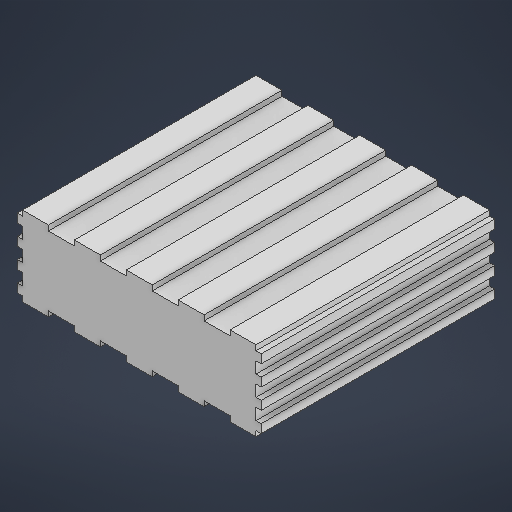
# Autodesk Inventor part: paredBase
Saved by Autodesk Inventor 2026 (Build 300175000, 175)
## iProperties
Created: 2026-04-21
Part Number: paredBase
Material: Generic
Document SubType Name: Modeling
Designer: juana
Density: 1 g/cm^3
Appearance: Default
Author: juana
Autodesk Inventor part; units mm, degrees
ref_plane "YZ Plane" through (0, 0, 0) normal (1, 0, 0) x (0, 1, 0)
ref_plane "XZ Plane" through (0, 0, 0) normal (0, 1, 0) x (-1, 0, 0)
ref_plane "XY Plane" through (0, 0, 0) normal (0, 0, 1) x (1, 0, 0)
sketch "Sketch1" plane through (0, 0, 0) normal (0, 0, 1) x (1, 0, 0)
  line L0 (0, 40) -> (135, 40)
  line L1 (135, 40) -> (135, 0)
  line L2 (135, 0) -> (0, 0)
  line L3 (0, 0) -> (0, 40)
  line L4 (-3, 40) -> (0, 40)
  line L5 (0, 40) -> (0, 35)
  line L6 (0, 35) -> (-3, 35)
  line L7 (-3, 35) -> (-3, 40)
  line L8 (-3, 28.35) -> (0, 28.35)
  line L9 (0, 28.35) -> (0, 23.35)
  line L10 (0, 23.35) -> (-3, 23.35)
  line L11 (-3, 23.35) -> (-3, 28.35)
  line L12 (-3, 16.7) -> (0, 16.7)
  line L13 (0, 16.7) -> (0, 11.7)
  line L14 (0, 11.7) -> (-3, 11.7)
  line L15 (-3, 11.7) -> (-3, 16.7)
  line L16 (135, 40) -> (138, 40)
  line L17 (138, 40) -> (138, 35)
  line L18 (138, 35) -> (135, 35)
  line L19 (135, 35) -> (135, 40)
  line L20 (135, 28.35) -> (138, 28.35)
  line L21 (138, 28.35) -> (138, 23.35)
  line L22 (138, 23.35) -> (135, 23.35)
  line L23 (135, 23.35) -> (135, 28.35)
  line L24 (135, 16.7) -> (138, 16.7)
  line L25 (138, 16.7) -> (138, 11.7)
  line L26 (138, 11.7) -> (135, 11.7)
  line L27 (135, 11.7) -> (135, 16.7)
  line L28 (0, 40) -> (15, 40)
  line L29 (15, 40) -> (15, 43)
  line L30 (15, 43) -> (0, 43)
  line L31 (0, 43) -> (0, 40)
  line L32 (30, 43) -> (30, 40)
  line L33 (30, 40) -> (45, 40)
  line L34 (45, 43) -> (30, 43)
  line L35 (45, 40) -> (45, 43)
  line L36 (60, 43) -> (60, 40)
  line L37 (60, 40) -> (75, 40)
  line L38 (75, 43) -> (60, 43)
  line L39 (75, 40) -> (75, 43)
  line L40 (90, 43) -> (90, 40)
  line L41 (90, 40) -> (105, 40)
  line L42 (105, 43) -> (90, 43)
  line L43 (105, 40) -> (105, 43)
  line L44 (120, 43) -> (120, 40)
  line L45 (120, 40) -> (135, 40)
  line L46 (135, 43) -> (120, 43)
  line L47 (135, 40) -> (135, 43)
  line L48 (0, 0) -> (0, -3)
  line L49 (0, -3) -> (15, -3)
  line L50 (15, 0) -> (0, 0)
  line L51 (15, -3) -> (15, 0)
  line L52 (30, 0) -> (30, -3)
  line L53 (30, -3) -> (45, -3)
  line L54 (45, 0) -> (30, 0)
  line L55 (45, -3) -> (45, 0)
  line L56 (60, 0) -> (60, -3)
  line L57 (60, -3) -> (75, -3)
  line L58 (75, 0) -> (60, 0)
  line L59 (75, -3) -> (75, 0)
  line L60 (90, 0) -> (90, -3)
  line L61 (90, -3) -> (105, -3)
  line L62 (105, 0) -> (90, 0)
  line L63 (105, -3) -> (105, 0)
  line L64 (120, 0) -> (120, -3)
  line L65 (120, -3) -> (135, -3)
  line L66 (135, 0) -> (120, 0)
  line L67 (135, -3) -> (135, 0)
  line L68 (-3, 5.05) -> (0, 5.05)
  line L69 (0, 5.05) -> (0, 0.05)
  line L70 (0, 0.05) -> (-3, 0.05)
  line L71 (-3, 0.05) -> (-3, 5.05)
  line L72 (135, 5.05) -> (138, 5.05)
  line L73 (138, 5.05) -> (138, 0.05)
  line L74 (138, 0.05) -> (135, 0.05)
  line L75 (135, 0.05) -> (135, 5.05)
  point P0 (15, 0)
  point P1 (30, 0)
  point P2 (45, 0)
  point P3 (60, 0)
  point P4 (75, 0)
  point P5 (90, 0)
  point P6 (105, 0)
  point P7 (120, 0)
  point P8 (135, 15)
  point P9 (105, 40)
  point P10 (75, 40)
  point P11 (45, 40)
  point P12 (15, 40)
  point P13 (0, 35)
  point P14 (0, 23.35)
  point P15 (0, 15)
  point P16 (135, 2)
  point P17 (0, 40)
  point P18 (0, 11.7)
  point P19 (0, 0)
  point P20 (0, 2)
  point P21 (135, 0)
  dimension "d0" = 40
  dimension "d1" = 135
  dimension "d2" = 3
  dimension "d3" = 5
  dimension "d6" = 11.65
  dimension "d9" = 138
  dimension "d12" = 3
  dimension "d13" = 15
  dimension "d16" = 30
  dimension "d19" = 43
  constraints: 152 end point, 6 parallel, 5 horizontal, 3 perpendicular, 2 vertical, 2 vertical alignment, 1 coincident, 1 horizontal alignment, 144 other
  measures "d0" distance of L0.end L1.end
  measures "d1" distance of L0.start L0.end
  measures "d2" distance of L4.start L4.end
  measures "d3" distance of L6.end L4.start
  measures "d6" distance of L0.start point (0, 28.35)
  measures "d9" distance of L0.start point (138, 40)
  measures "d12" distance of L30.end L4.end
  measures "d13" distance of L29.end L30.end
  measures "d16" distance of L0.start point (30, 40)
  measures "d19" distance of L0.start point (0, -3)
extrude "Extrusion1" add sketch "Sketch1" along normal blind 135
equation "\"d22\" = d1"
body "Solid1"
